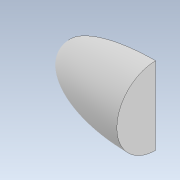
# Autodesk Inventor part: Расчетная область
Saved by Autodesk Inventor 2020 (Build 240168000, 168)
## iProperties
Created: 2023-04-25
Part Number: Расчетная область
Material: Типовые
Document SubType Name: Modeling
Designer: user
Density: 1 g/cm^3
Appearance: По умолчанию
Mass: 593.319 g
Surface Area: 491.974 cm^2
Volume: 593.319 cm^3
Author: user
Autodesk Inventor part; units mm, degrees
ref_plane "YZ Plane" through (0, 0, 0) normal (1, 0, 0) x (0, 1, 0)
ref_plane "XZ Plane" through (0, 0, 0) normal (0, 1, 0) x (-1, 0, 0)
ref_plane "XY Plane" through (0, 0, 0) normal (0, 0, 1) x (1, 0, 0)
sketch "Эскиз1" plane through (0, 0, 0) normal (0, 0, 1) x (1, 0, 0)
  line L0 (0, 0) -> (342.9, 0)
  line L1 (172.4011, 28.562) -> (172.4011, 0)
  line L2 (172.4011, 28.562) -> (286.7011, 28.562)
  line L3 (286.7011, 28.562) -> (286.7011, 0)
  line L4 (286.7011, 28.562) -> (342.9, 21.6616)
  line L5 (342.9, 21.6616) -> (342.9, 0)
  arc A0 (172.4011, 28.562) -> (0, 0) centre (261.9756, -1046.7023) ccw
  line L6 (286.7011, 0) -> (286.7011, -1353.3259)
  line L7 (342.9, 0) -> (342.9, -1353.3129)
  point P0 (172.4, 28.5619)
  dimension "d0" = 342.9
  dimension "d3" = 114.3
  dimension "d4" = 7
  dimension "d5" = 1046.7023
  dimension "d6" = 261.9756
  constraints: 16 end point, 3 vertical, 2 horizontal, 2 perpendicular, 2 point on circle, 2 point on line, 1 centre point, 1 coincident
  measures "d0" distance of L0.start L0.end
  measures "d3" distance of L1.start L2.end
  measures "d4" angle of L4 L2
  measures "d5" distance from line of L0 point (261.976, -1046.702)
  measures "d6" horizontal distance of point (261.976, -1046.702) L0.start
revolve "Вращение1" add sketch "Эскиз1" angle 360 about axis through (0, 0, 0) along (1, 0, 0)
sketch "Эскиз2" plane through (0, 0, 0) normal (0, 0, 1) x (1, 0, 0)
  ellipse E0 centre (692.9, 0) end of major axis (-500, 0) minor radius 500
  line L0 (342.9, -21.6616) -> (342.9, 21.6616) projected
  line L1 (692.9, 500) -> (692.9, 0)
  line L2 (692.9, 0) -> (692.9, -500)
  line L3 (-500, 0) -> (692.9, 0)
  point P0 (0, 0)
  dimension "d8" = 342.9
  dimension "d9" = 500
  dimension "d10" = 500
  dimension "d11" = 350
  constraints: 6 end point, 1 horizontal, 1 point on line, 1 vertical, 5 other
  measures "d8" distance from line of point (0, 0) L0
  measures "d9" distance of L3.start point (0, 0)
  measures "d10" distance of L1.start L1.end
  measures "d11" distance from line of L1.end L0
revolve "Вращение2" add sketch "Эскиз2" angle 180 about axis through (-500, 0, 0) along (1, 0, 0) separate body contours E0 L1 L3
combine bodies "Комбинировать1" operation type subtract main body 2 bodies to subtract 1
